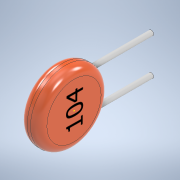
# Autodesk Inventor part: cap334
Saved by Autodesk Inventor 2020 (Build 240168000, 168)
## iProperties
Created: 2021-10-19
Part Number: cap334
Material: Genérico
Document SubType Name: Modeling
Designer: DANIEL
Density: 1 g/cm^3
Appearance: Valor por defecto
Author: DANIEL
Autodesk Inventor part; units mm, degrees
ref_plane "YZ Plane" through (0, 0, 0) normal (1, 0, 0) x (0, 1, 0)
ref_plane "XZ Plane" through (0, 0, 0) normal (0, 1, 0) x (-1, 0, 0)
sketch "Boceto1" plane through (0, 0, 0) normal (1, 0, 0) x (0, 1, 0)
  circle A0 centre (0, 0) radius 2.15
  dimension "d0" = 4.3
  constraints: 1 centre point, 1 coincident
  measures "d0" diameter of A0
extrude "Extrusión1" add sketch "Boceto1" along normal mid plane 1.2
fillet "Empalme1" radius 0.5 1 edges at (0.6, -2.15, 0)
fillet "Empalme2" radius 0.5 1 edges at (-0.6, -2.15, 0)
sketch "Boceto2" plane through (-0.6, 0, 0) normal (-1, 0, 0) x (0, 0, 1)
  line L0 (-0.4973, -1.1141) -> (-0.471, 1.1369) construction
  line L1 (-0.471, 1.1369) -> (0.5703, 1.1247) construction
  line L2 (0.5703, 1.1247) -> (0.544, -1.1263) construction
  line L3 (0.544, -1.1263) -> (-0.4973, -1.1141) construction
  line L4 (-0.4973, -1.1141) -> (-0.471, 1.1369) construction
  line L5 (-0.471, 1.1369) -> (0.5703, 1.1247) construction
  line L6 (0.5703, 1.1247) -> (0.544, -1.1263) construction
  line L7 (0.544, -1.1263) -> (-0.4973, -1.1141) construction
  line L8 (-0.4973, -1.1141) -> (-0.471, 1.1369) construction
  line L9 (-0.471, 1.1369) -> (0.5703, 1.1247) construction
  line L10 (0.5703, 1.1247) -> (0.544, -1.1263) construction
  line L11 (0.544, -1.1263) -> (-0.4973, -1.1141) construction
  line L12 (-0.4973, -1.1141) -> (-0.471, 1.1369) construction
  line L13 (-0.471, 1.1369) -> (0.5703, 1.1247) construction
  line L14 (0.5703, 1.1247) -> (0.544, -1.1263) construction
  line L15 (0.544, -1.1263) -> (-0.4973, -1.1141) construction
  line L16 (0.5613, 1.1178) -> (0.5386, -1.1333) construction
  line L17 (0.5386, -1.1333) -> (-0.5027, -1.1227) construction
  line L18 (-0.5027, -1.1227) -> (-0.4799, 1.1284) construction
  line L19 (-0.4799, 1.1284) -> (0.5613, 1.1178) construction
  point P0 (0, 0)
  constraints: 6 other
sketch "Boceto3" plane through (0.6, 0, 0) normal (1, 0, 0) x (0, 0, -1)
  line L0 (-0.4973, -1.1141) -> (-0.471, 1.1369) construction
  line L1 (-0.471, 1.1369) -> (0.5703, 1.1247) construction
  line L2 (0.5703, 1.1247) -> (0.544, -1.1263) construction
  line L3 (0.544, -1.1263) -> (-0.4973, -1.1141) construction
  point P0 (0, 0)
  constraints: 2 other
ref_plane "Plano de trabajo1" through (0, 0, -1.3) normal (0, 0, 1) x (1, 0, 0)
sketch "Boceto4" plane through (0, 0, -1.3) normal (0, 0, 1) x (1, 0, 0)
  line L0 (0.1, -2.15) -> (0.1, 2.15) projected
  line L1 (0.6, 1.65) -> (0.6, -1.65) projected
  line L2 (-0.1, 2.15) -> (-0.1, -2.15) projected
  line L3 (-0.6, -1.65) -> (-0.6, 1.65) projected
  line L4 (0.1, -2.15) -> (0.1, 2.15) projected
  line L5 (-0.1, 2.15) -> (-0.1, -2.15) projected
  circle A0 centre (0, -1.0922) radius 0.15
  circle A1 centre (0, 1.152) radius 0.15
  point P0 (0, 0)
  dimension "d7" = 0.3
  dimension "d8" = 0.3
  constraints: 2 centre point
  measures "d7" diameter of A0
  measures "d8" diameter of A1
extrude "Extrusión2" add sketch "Boceto4" against normal blind 4 contours A0 L2 L0 | L0 A0 | A0 L2 | A1 L2 L0 | L0 A1 | A1 L2
